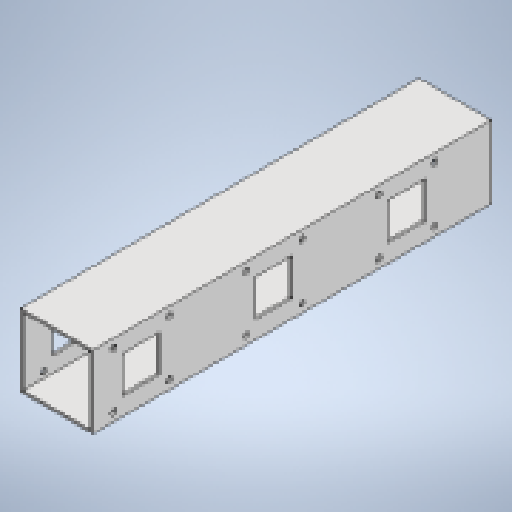
# Autodesk Inventor part: PRS 940-55 (fds) main way tube
Saved by Autodesk Inventor 2025.3 (Build 293356030, 356C)
## iProperties
Created: 2025-06-24
Part Number: PRS 940-55 (fds) main way tube
Material: Stainless Steel
Document SubType Name: Modeling
Designer: admin
Mass: 1762.25 g
Surface Area: 2283.33 cm^2
Volume: 220.281 cm^3
Density: 8 g/cm^3
Sheet Metal Rule: AISI304 2mm Die16
Sheet Metal Width: 0.000 mm
Sheet Metal Length: 0.000 mm
Sheet Metal Area: 0.000 mm^2
Appearance: Default
Author: user
Autodesk Inventor part; units mm, degrees
ref_plane "YZ Plane" through (0, 0, 0) normal (1, 0, 0) x (0, 1, 0)
ref_plane "XZ Plane" through (0, 0, 0) normal (0, 1, 0) x (-1, 0, 0)
ref_plane "XY Plane" through (0, 0, 0) normal (0, 0, 1) x (1, 0, 0)
sketch "Sketch9" plane through (0, 0, 0) normal (0, 1, 0) x (-1, 0, 0)
  line L0 (30, 30) -> (-30, 30)
  line L1 (-30, 30) -> (-30, -30)
  line L2 (-30, -30) -> (30, -30)
  line L3 (30, -30) -> (30, 30)
  line L4 (30, 30) -> (-30, -30) construction
  line L5 (-30, 30) -> (30, -30) construction
  line L6 (-28, 28) -> (28, 28)
  line L7 (28, 28) -> (28, -28)
  line L8 (28, -28) -> (-28, -28)
  line L9 (-28, -28) -> (-28, 28)
  point P0 (0, 0)
  dimension "d172" = 60
  dimension "d173" = 60
  dimension "d174" = 2
  constraints: 20 end point, 4 parallel, 2 midpoint, 2 perpendicular, 1 horizontal, 3 other
  measures "d172" distance of L2.end L1.end
  measures "d173" distance of L0.end L1.end
  measures "d174" distance between parallel lines of L0 L6
extrude "Extrusion3" add sketch "Sketch9" against normal blind 330
sketch "Sketch10" plane through (0, 0, 0) normal (1, 0, 0) x (0, 1, 0)
  line L0 (0, 30) -> (0, -30) construction
  line L1 (0, 30) -> (-330, 30) construction
  line L2 (-330, -30) -> (-330, 30) construction
  line L3 (0, -30) -> (-330, -30) construction
  line L4 (0, 0) -> (40, 0)
  line L5 (-85.25, -15.25) -> (-85.25, 15.25)
  line L6 (-85.25, 15.25) -> (-54.75, 15.25)
  line L7 (-54.75, 15.25) -> (-54.75, -15.25)
  line L8 (-54.75, -15.25) -> (-85.25, 15.25) construction
  line L9 (-85.25, -15.25) -> (-54.75, 15.25) construction
  circle A0 centre (-93, 23) radius 2.5
  circle A1 centre (-47, 23) radius 2.5
  line L10 (-85.25, -15.25) -> (-93, -23) construction
  circle A2 centre (-47, -23) radius 2.5
  circle A3 centre (-93, -23) radius 2.5
  circle A4 centre (-70, 0) radius 32.5269 construction
  line L11 (-54.75, -15.25) -> (-85.25, -15.25)
  line L12 (-44.5, -25.5) -> (-95.5, -25.5) construction
  line L13 (-95.5, -25.5) -> (-95.5, 25.5) construction
  line L14 (-95.5, 25.5) -> (-44.5, 25.5) construction
  line L15 (-44.5, 25.5) -> (-44.5, -25.5) construction
  line L16 (-44.5, -25.5) -> (-95.5, 25.5) construction
  line L17 (-95.5, -25.5) -> (-44.5, 25.5) construction
  line L18 (-70, 37.0891) -> (-70, 0) construction
  circle A5 centre (-93, 23) radius 10.9602 construction
  point P0 (-391.3995, 90.0207)
  point P1 (-386.6495, 165.0207)
  dimension "d191" = 21.9203
  dimension "d181" = 40
  dimension "d187" = 30.5
  dimension "d188" = 30.5
  dimension "d189" = 5
  dimension "d190" = 51
  dimension "d192" = 110
  dimension "d196" = 46
  constraints: 32 end point, 6 point on line, 5 centre point, 5 midpoint, 4 parallel, 4 point on circle, 3 equal radius, 3 horizontal, 2 coincident, 2 perpendicular, 1 tangent, 1 vertical, 3 other
  measures "d181" distance of L4.start L4.end
  measures "d187" distance of L7.end L5.start
  measures "d188" distance of L5.start L5.end
  measures "d189" diameter of A2
  measures "d190" distance of L13.start L13.end
  measures "d192" distance of L4.end L18.end
  measures "d196" distance of A0.centre A1.centre
extrude "Extrusion4" cut sketch "Sketch10" along normal through all both and the other way through all
pattern_linear "Rectangular Pattern4" count 3 spacing 110 along (0, -1, 0) of "Extrusion4"
body "Solid4"
